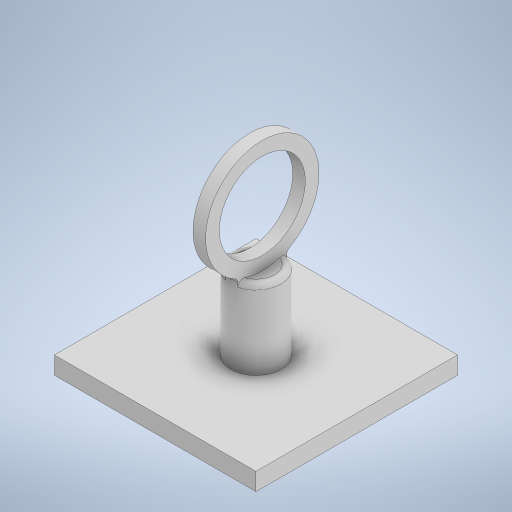
# Autodesk Inventor part: Base para el Ensamble
Saved by Autodesk Inventor 2024.2 (Build 282272000, 272)
## iProperties
Created: 2024-03-31
Part Number: Base para el Ensamble
Material: Generic
Document SubType Name: Modeling
Designer: Josh Juárez
Density: 1 g/cm^3
Appearance: Default
Author: Josh Juárez
Autodesk Inventor part; units mm, degrees
ref_plane "YZ Plane" through (0, 0, 0) normal (1, 0, 0) x (0, 1, 0)
ref_plane "XZ Plane" through (0, 0, 0) normal (0, 1, 0) x (-1, 0, 0)
ref_plane "XY Plane" through (0, 0, 0) normal (0, 0, 1) x (1, 0, 0)
sketch "Sketch1" plane through (0, 0, 0) normal (1, 0, 0) x (0, 1, 0)
  circle A0 centre (0, 0) radius 17.07
  circle A1 centre (0, 0) radius 22.5
  dimension "d0" = 34.14
  dimension "d1" = 45
  constraints: 2 centre point, 2 coincident
  measures "d0" diameter of A0
  measures "d1" diameter of A1
extrude "Extrusion1" add sketch "Sketch1" along normal blind 5
ref_plane "Work Plane1" through (2.5, 0, 0) normal (1, 0, 0) x (0, 0, -1)
sketch "Sketch4" plane through (2.5, 0, 0) normal (1, 0, 0) x (0, 0, -1)
  circle A0 centre (0, 0) radius 22.5 projected
  line L0 (0, -22.5) -> (0, -52.5)
  line L1 (0, -52.5) -> (10, -52.5)
  line L2 (10, -52.5) -> (10, -20.1556)
  arc A1 (0, -22.5) -> (10, -20.1556) centre (0, 0) ccw
  line L3 (0, -67.5) -> (0, 37.5) projected
  dimension "d11" = 30
  dimension "d12" = 10
  constraints: 6 end point, 4 point on circle, 2 perpendicular, 1 centre point, 1 concentric, 1 vertical
  measures "d11" distance of L0.start L0.end
  measures "d12" distance of L0.end L1.end
revolve "Revolution1" add sketch "Sketch4" angle 360 about axis through (2.5, -10, 0) along (0, 1, 0) contours A0 L2 L1 L0
fillet "Fillet1" radius 2 6 edges at (-7.5, -20.1556, 0) (12.5, -20.1556, 0) (1.2426, -20.1948, -9.9206) (3.7574, -20.1948, -9.9206) (1.2426, -20.1948, 9.9206) (3.7574, -20.1948, 9.9206)
sketch "Sketch5" plane through (2.5, -52.5, 0) normal (0, -1, 0) x (1, 0, 0)
  line L0 (40, 0) -> (40, -40)
  line L1 (40, -40) -> (-40, -40)
  line L2 (-40, -40) -> (-40, 40)
  line L3 (-40, 40) -> (40, 40)
  line L4 (40, 40) -> (40, 0)
  point P0 (-2.5, 0)
  dimension "d18" = 40
  dimension "d19" = 80
  dimension "d20" = 80
  dimension "d21" = 80
  constraints: 10 end point, 2 perpendicular, 1 point on line, 1 vertical
  measures "d18" distance of L0.start L0.end
  measures "d19" distance of L0.end L1.end
  measures "d20" distance of L1.end L2.end
  measures "d21" distance of L2.end L3.end
extrude "Extrusion2" add sketch "Sketch5" along normal blind 7
body "Solid1"
